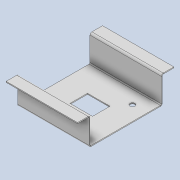
# Autodesk Inventor part: Base vacuometro
Saved by Autodesk Inventor 2021 (Build 250183000, 183)
## iProperties
Created: 2021-06-01
Part Number: Base vacuometro
Material: Genérico
Document SubType Name: Chapa
Designer: Admin
Density: 1 g/cm^3
Sheet Metal Rule: Por defecto_mm
Appearance: Valor por defecto
Flat Pattern Width: 5.7 cm
Flat Pattern Length: 11.7236 cm
Flat Pattern Area: 66.8247 cm^2
Sheet Metal Width: 57,000 mm
Sheet Metal Length: 117,236 mm
Sheet Metal Area: 6682,470 mm^2
Author: Admin
Autodesk Inventor part; units mm, degrees
ref_plane "YZ Plane" through (0, 0, 0) normal (1, 0, 0) x (0, 1, 0)
ref_plane "XZ Plane" through (0, 0, 0) normal (0, 1, 0) x (-1, 0, 0)
ref_plane "XY Plane" through (0, 0, 0) normal (0, 0, 1) x (1, 0, 0)
sketch "Boceto1" plane through (0, 0, 0) normal (0, 1, 0) x (-1, 0, 0)
  line L0 (0, 0) -> (57, 0)
  line L1 (57, 0) -> (57, -57)
  line L2 (57, -57) -> (0, -57)
  line L3 (0, -57) -> (0, 0)
  dimension "d0" = 57
  dimension "d1" = 57
  measures "d0" distance of L1.end L2.end
  measures "d1" distance of L0.end L1.end
extrude "Placa1" add sketch "Boceto1" along normal blind 0.76
sketch "Boceto2" plane through (-57, 0.76, -57) normal (0, 0, -1) x (-1, 0, 0)
  line L0 (-57, 0) -> (0, 0)
  line L1 (0, 0) -> (0, 21.24)
  line L2 (0, 21.24) -> (-57, 21.24)
  line L3 (-57, 21.24) -> (-57, 0)
  constraints: 6 end point, 1 horizontal, 1 perpendicular, 1 vertical
edge flange "Pestaña1" height 22 angle 90 thickness 0.76 bend radius 0.76 thickness toward (0, 0, -1) relief straight relief width 0.76 relief depth 0.38 corner gap 0.76 corner form 0 edges at (-28.5, 0.76, -57) (-28.5, 0.76, 0) wall of the first edge with corners at (0, 0.76, -57) (-57, 0.76, -57) (-57, 22, -57) (0, 22, -57)
bend "Doblez1"
corner "Esquina1"
sketch "Boceto3" plane through (-57, 21.24, -57) normal (0, 1, 0) x (-1, 0, 0)
  line L0 (-57, 0) -> (0, 0)
  line L1 (0, 0) -> (0, 10)
  line L2 (0, 10) -> (-57, 10)
  line L3 (-57, 10) -> (-57, 0)
  constraints: 6 end point, 1 horizontal, 1 perpendicular, 1 vertical
edge flange "Pestaña2" height 10 angle 90 thickness 0.76 bend radius 0.76 thickness toward (0, 1, 0) relief straight relief width 0.76 relief depth 0.38 corner gap 0.76 corner form 0 edges at (-28.5, 22, -57) (-28.5, 22, 0) wall of the first edge with corners at (0, 21.24, -57) (-57, 21.24, -57) (-57, 21.24, -67) (0, 21.24, -67)
bend "Doblez2"
corner "Esquina2"
sketch "Boceto6" plane through (0, 0, 0) normal (0, -1, 0) x (1, 0, 0)
  line L0 (0, -56.24) -> (0, -0.76) projected
  line L1 (-57, -0.76) -> (-57, -56.24) projected
  line L2 (0, -56.24) -> (-57, -56.24) projected
  line L3 (-37.5, -21.5) -> (-19.5, -21.5)
  line L4 (-19.5, -21.5) -> (-19.5, -35.5)
  line L5 (-19.5, -35.5) -> (-37.5, -35.5)
  line L6 (-37.5, -35.5) -> (-37.5, -21.5)
  line L7 (-37.5, -21.5) -> (-19.5, -35.5) construction
  line L8 (-19.5, -21.5) -> (-37.5, -35.5) construction
  point P0 (0, 0)
  constraints: 12 end point, 2 parallel, 1 horizontal, 1 perpendicular
extrude "Extrusión2" cut sketch "Boceto6" against normal through all
sketch "Boceto7" plane through (0, 0, 0) normal (0, -1, 0) x (1, 0, 0)
  circle A0 centre (-45.4706, -11.5294) radius 2 projected
  circle A1 centre (-11.5294, -45.4706) radius 2 projected
  point P0 (0, 0)
extrude "Extrusión3" cut sketch "Boceto7" against normal through all
equation "\"d2\" = Grosor"
equation "\"d3\" = Anchura_desahogo_plegado"
equation "\"d4\" = Profundidad_desahogo_plegado"
equation "\"d5\" = Remanente_mínimo"
equation "\"d6\" = Radiodetransición"
equation "\"d9\" = Radio_pliegue"
equation "\"d10\" = Tamaño_destalonado"
equation "\"d11\" = TamañoSeparación"
equation "\"d12\" = Tamaño_de_radio_de_Jacobi"
equation "\"d13\" = Anchura_desahogo_plegado"
equation "\"d14\" = Profundidad_desahogo_plegado"
equation "\"d15\" = Remanente_mínimo"
equation "\"d16\" = Radiodetransición"
equation "\"d19\" = Radio_pliegue"
equation "\"d20\" = Tamaño_destalonado"
equation "\"d21\" = TamañoSeparación"
equation "\"d22\" = Tamaño_de_radio_de_Jacobi"
equation "\"Radio_pliegue\" = Grosor"
equation "\"Anchura_desahogo_plegado\" = Grosor"
equation "\"Profundidad_desahogo_plegado\" = 0.5 * Grosor"
equation "\"Tamaño_destalonado\" = 4 * Grosor"
equation "\"Remanente_mínimo\" = 2 * Grosor"
equation "\"Radiodetransición\" = Radio_pliegue"
equation "\"Tamaño_de_radio_de_Jacobi\" = Radio_pliegue"
equation "\"TamañoSeparación\" = Grosor"
equation "\"Grosor\" = 0.76"
